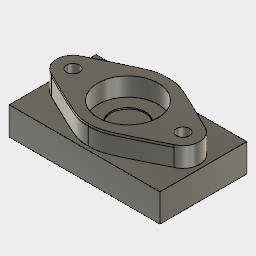
bearings-shredder v5 (Autodesk Fusion 360 design; units mm, degrees)
Autodesk Fusion 360 part; units mm, degrees
box "BoxPrimitive1" add length 68 width 118 height 22 placed x (0, 1, 0) y (-1, 0, 0) z (0, 0, 1) at (118, 0, 0) makes body 1
sketch "Sketch2" plane through (0, 0, 22) normal (0, 0, 1) x (-1, 0, 0)
  line L0 (-118, -68) -> (0, -68)
  line L1 (0, -68) -> (0, 0)
  line L2 (0, 0) -> (-118, 0)
  line L3 (-118, 0) -> (-118, -68)
  line L4 (0, -68) -> (-118, 0)
  line L5 (-118, -68) -> (0, 0)
  circle A0 centre (-59, -34) radius 23.5
extrude "Extrude1" cut sketch "Sketch2" against normal blind 21 contours L4 L5 A0 | L4 L5 A0 | L4 L5 A0 | L4 L5 A0 bodies 1
sketch "Sketch3" plane through (0, 0, 22) normal (0, 0, 1) x (-1, 0, 0)
  circle A0 centre (-59, -34) radius 23.5
  line L0 (-118, -68) -> (0, -68)
  line L1 (0, -68) -> (0, 0)
  line L2 (0, 0) -> (-118, 0)
  line L3 (-118, 0) -> (-118, -68)
  circle A1 centre (-59, -34) radius 13.5
  dimension "d9" = 27
  measures "d9" diameter of A1
extrude "Extrude2" cut sketch "Sketch3" against normal blind 22 contours A1 bodies 1
sketch "Sketch4" plane through (0, 0, 22) normal (0, 0, 1) x (-1, 0, 0)
  circle A0 centre (-59, -34) radius 23.5
  line L0 (-118, -68) -> (0, -68)
  line L1 (0, -68) -> (0, 0)
  line L2 (0, 0) -> (-118, 0)
  line L3 (-118, 0) -> (-118, -68)
  line L4 (-59, -34) -> (-59, -65)
  line L5 (-59, -34) -> (-90, -34)
  line L6 (-59, -34) -> (-59, -3)
  line L7 (-59, -34) -> (-112, -34)
  line L8 (-59, -34) -> (-6, -34)
  line L9 (-6, -34) -> (-26, -34)
  line L10 (-112, -34) -> (-92, -34)
  line L11 (-6, -34) -> (-16, -34)
  line L12 (-112, -34) -> (-102, -34)
  circle A1 centre (-16, -34) radius 13
  circle A2 centre (-59, -34) radius 31
  circle A3 centre (-102, -34) radius 13
  spline S0 degree 2 poles (-59, -65) (-49.9968, -65) (-11.1653, -46.0676) knots 0 0 0 5.176536 5.176536 5.176536 weights 1 3 1
  spline S1 degree 2 poles (-59, -3) (-49.9644, -3) (-11.1653, -21.9324) knots 0 0 0 5.176727 5.176727 5.176727 weights 1 3 1
  spline S2 degree 2 poles (-59, -65) (-68.866, -65) (-107, -46) knots 0 0 0 5.199566 5.199566 5.199566 weights 1 3 1
  spline S3 degree 2 poles (-59, -3) (-68.866, -3) (-107, -22) knots 0 0 0 5.199566 5.199566 5.199566 weights 1 3 1
  dimension "d14" = 31
  dimension "d21" = 26
  dimension "d22" = 26
  measures "d14" distance of A0.centre L6.end
  measures "d21" diameter of A1
  measures "d22" diameter of A3
cylinder "CylinderPrimitive1" cut diameter 10 height -22 placed x (1, 0, 0) y (0, 1, 0) z (0, 0, 1) at (16, 34, 22) bodies 1
cylinder "CylinderPrimitive2" cut diameter 10 height -22 placed x (1, 0, 0) y (0, 1, 0) z (0, 0, 1) at (102, 34, 22) bodies 1
box "BoxPrimitive2" add length 68 width 118 height -22 placed x (0, 1, 0) y (-1, 0, 0) z (0, 0, 1) at (118, 0, 22) separate body makes body 2
extrude "Extrude3" cut sketch "Sketch4" against normal blind 22 bodies 1
extrude "Extrude4" cut 1 faces at (87.5583, 16.7442, 22) along direction (0, 0, -1) blind 7 on bodies 1 bodies 1
extrude "Extrude5" add 1 faces at (38.9711, 32.1618, 1) along direction (0, 0, 1) blind 2 on bodies 1 bodies 1
copy_body "CopyPasteBodies1" bodies 2 makes body 3
move_body "Move1" bodies 3 to x (1, 0, 0) y (0, 1, 0) z (0, 0, 1) at (0, 0, -22)
combine "Combine1" operation add target body 1 tool bodies 3
extrude "Extrude6" cut 1 faces at (87.5583, 16.7442, 15) along direction (0, 0, -1) blind 1.5 on bodies 1 bodies 1
extrude "Extrude7" cut 1 faces at (38.9711, 32.1618, 3) along direction (0, 0, -1) blind 2 on bodies 1 bodies 1
extrude "Extrude8" add 1 faces at (87.5583, 16.7442, 13.5) along direction (0, 0, 1) blind 0.9 on bodies 1 bodies 1
extrude "Extrude9" add 1 faces at (87.5583, 16.7442, 14.4) along direction (0, 0, 1) blind 1 on bodies 1 bodies 1
box "BoxPrimitive5" add length 68 width 118 height 15.3 placed x (0, 1, 0) y (-1, 0, 0) z (0, 0, 1) at (118, 0, 0) separate body makes body 4
hidden bodies 2 4
